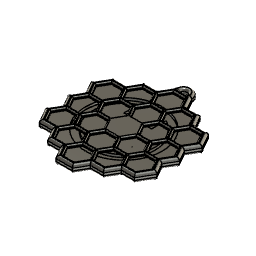
Base-v01 v7 (Autodesk Fusion 360 design; units mm, degrees)
Autodesk Fusion 360 part; units mm, degrees
sketch "Skizze1" plane through (0, 0, 0) normal (0, 0, 1) x (1, 0, 0)
  line L0 (2.5981, -13.5) -> (5.1962, -9) construction
  line L1 (5.1962, -9) -> (2.5981, -4.5) construction
  line L2 (2.5981, -4.5) -> (-2.5981, -4.5) construction
  line L3 (-2.5981, -4.5) -> (-5.1962, -9) construction
  line L4 (-5.1962, -9) -> (-2.5981, -13.5) construction
  line L5 (-2.5981, -13.5) -> (2.5981, -13.5) construction
  line L6 (-2.5981, -4.5) -> (-5.1962, 0) construction
  line L7 (-5.1962, 0) -> (-10.3923, 0) construction
  line L8 (-10.3923, 0) -> (-12.9904, -4.5) construction
  line L9 (-12.9904, -4.5) -> (-10.3923, -9) construction
  line L10 (-10.3923, -9) -> (-5.1962, -9) construction
  line L11 (-5.1962, -9) -> (-2.5981, -4.5) construction
  line L12 (-5.1962, -9) -> (-10.3923, -9) construction
  line L13 (-10.3923, -9) -> (-12.9904, -13.5) construction
  line L14 (-12.9904, -13.5) -> (-10.3923, -18) construction
  line L15 (-10.3923, -18) -> (-5.1962, -18) construction
  line L16 (-5.1962, -18) -> (-2.5981, -13.5) construction
  line L17 (-2.5981, -13.5) -> (-5.1962, -9) construction
  line L18 (12.9904, -13.5) -> (10.3923, -9) construction
  line L19 (10.3923, -9) -> (5.1962, -9) construction
  line L20 (5.1962, -9) -> (2.5981, -13.5) construction
  line L21 (2.5981, -13.5) -> (5.1962, -18) construction
  line L22 (5.1962, -18) -> (10.3923, -18) construction
  line L23 (10.3923, -18) -> (12.9904, -13.5) construction
  line L24 (12.9904, -4.5) -> (10.3923, 0) construction
  line L25 (10.3923, 0) -> (5.1962, 0) construction
  line L26 (5.1962, 0) -> (2.5981, -4.5) construction
  line L27 (2.5981, -4.5) -> (5.1962, -9) construction
  line L28 (5.1962, -9) -> (10.3923, -9) construction
  line L29 (10.3923, -9) -> (12.9904, -4.5) construction
  line L30 (20.7846, 0) -> (18.1865, 4.5) construction
  line L31 (18.1865, 4.5) -> (12.9904, 4.5) construction
  line L32 (12.9904, 4.5) -> (10.3923, 0) construction
  line L33 (10.3923, 0) -> (12.9904, -4.5) construction
  line L34 (12.9904, -4.5) -> (18.1865, -4.5) construction
  line L35 (18.1865, -4.5) -> (20.7846, 0) construction
  line L36 (10.3923, -9) -> (12.9904, -13.5) construction
  line L37 (12.9904, -13.5) -> (18.1865, -13.5) construction
  line L38 (18.1865, -13.5) -> (20.7846, -9) construction
  line L39 (20.7846, -9) -> (18.1865, -4.5) construction
  line L40 (18.1865, -4.5) -> (12.9904, -4.5) construction
  line L41 (12.9904, -4.5) -> (10.3923, -9) construction
  line L42 (-5.1962, 0) -> (-2.5981, -4.5) construction
  line L43 (-2.5981, -4.5) -> (2.5981, -4.5) construction
  line L44 (2.5981, -4.5) -> (5.1962, 0) construction
  line L45 (5.1962, 0) -> (2.5981, 4.5) construction
  line L46 (2.5981, 4.5) -> (-2.5981, 4.5) construction
  line L47 (-2.5981, 4.5) -> (-5.1962, 0) construction
  line L48 (-10.3923, -27) -> (-5.1962, -27) construction
  line L49 (-5.1962, -27) -> (-2.5981, -22.5) construction
  line L50 (-2.5981, -22.5) -> (-5.1962, -18) construction
  line L51 (-5.1962, -18) -> (-10.3923, -18) construction
  line L52 (-10.3923, -18) -> (-12.9904, -22.5) construction
  line L53 (-12.9904, -22.5) -> (-10.3923, -27) construction
  line L54 (10.3923, -36) -> (12.9904, -31.5) construction
  line L55 (12.9904, -31.5) -> (10.3923, -27) construction
  line L56 (10.3923, -27) -> (5.1962, -27) construction
  line L57 (5.1962, -27) -> (2.5981, -31.5) construction
  line L58 (2.5981, -31.5) -> (5.1962, -36) construction
  line L59 (5.1962, -36) -> (10.3923, -36) construction
  line L60 (2.5981, -31.5) -> (5.1962, -27) construction
  line L61 (5.1962, -27) -> (2.5981, -22.5) construction
  line L62 (2.5981, -22.5) -> (-2.5981, -22.5) construction
  line L63 (-2.5981, -22.5) -> (-5.1962, -27) construction
  line L64 (-5.1962, -27) -> (-2.5981, -31.5) construction
  line L65 (-2.5981, -31.5) -> (2.5981, -31.5) construction
  line L66 (28.5788, -13.5) -> (25.9808, -9) construction
  line L67 (25.9808, -9) -> (20.7846, -9) construction
  line L68 (20.7846, -9) -> (18.1865, -13.5) construction
  line L69 (18.1865, -13.5) -> (20.7846, -18) construction
  line L70 (20.7846, -18) -> (25.9808, -18) construction
  line L71 (25.9808, -18) -> (28.5788, -13.5) construction
  line L72 (12.9904, -22.5) -> (10.3923, -18) construction
  line L73 (10.3923, -18) -> (5.1962, -18) construction
  line L74 (5.1962, -18) -> (2.5981, -22.5) construction
  line L75 (2.5981, -22.5) -> (5.1962, -27) construction
  line L76 (5.1962, -27) -> (10.3923, -27) construction
  line L77 (10.3923, -27) -> (12.9904, -22.5) construction
  line L78 (18.1865, -22.5) -> (12.9904, -22.5) construction
  line L79 (12.9904, -22.5) -> (10.3923, -27) construction
  line L80 (10.3923, -27) -> (12.9904, -31.5) construction
  line L81 (12.9904, -31.5) -> (18.1865, -31.5) construction
  line L82 (18.1865, -31.5) -> (20.7846, -27) construction
  line L83 (20.7846, -27) -> (18.1865, -22.5) construction
  line L84 (10.3923, 9) -> (5.1962, 9) construction
  line L85 (5.1962, 9) -> (2.5981, 4.5) construction
  line L86 (2.5981, 4.5) -> (5.1962, 0) construction
  line L87 (5.1962, 0) -> (10.3923, 0) construction
  line L88 (10.3923, 0) -> (12.9904, 4.5) construction
  line L89 (12.9904, 4.5) -> (10.3923, 9) construction
  line L90 (18.1865, -13.5) -> (12.9904, -13.5) construction
  line L91 (12.9904, -13.5) -> (10.3923, -18) construction
  line L92 (10.3923, -18) -> (12.9904, -22.5) construction
  line L93 (12.9904, -22.5) -> (18.1865, -22.5) construction
  line L94 (18.1865, -22.5) -> (20.7846, -18) construction
  line L95 (20.7846, -18) -> (18.1865, -13.5) construction
  line L96 (25.9808, 0) -> (20.7846, 0) construction
  line L97 (20.7846, 0) -> (18.1865, -4.5) construction
  line L98 (18.1865, -4.5) -> (20.7846, -9) construction
  line L99 (20.7846, -9) -> (25.9808, -9) construction
  line L100 (25.9808, -9) -> (28.5788, -4.5) construction
  line L101 (28.5788, -4.5) -> (25.9808, 0) construction
  line L102 (2.5981, -22.5) -> (5.1962, -18) construction
  line L103 (5.1962, -18) -> (2.5981, -13.5) construction
  line L104 (2.5981, -13.5) -> (-2.5981, -13.5) construction
  line L105 (-2.5981, -13.5) -> (-5.1962, -18) construction
  line L106 (-5.1962, -18) -> (-2.5981, -22.5) construction
  line L107 (-2.5981, -22.5) -> (2.5981, -22.5) construction
  line L108 (28.5788, -22.5) -> (25.9808, -18) construction
  line L109 (25.9808, -18) -> (20.7846, -18) construction
  line L110 (20.7846, -18) -> (18.1865, -22.5) construction
  line L111 (18.1865, -22.5) -> (20.7846, -27) construction
  line L112 (20.7846, -27) -> (25.9808, -27) construction
  line L113 (25.9808, -27) -> (28.5788, -22.5) construction
  line L114 (5.5426, 0.6) -> (10.0459, 0.6)
  line L115 (10.0459, 0.6) -> (12.2976, 4.5)
  line L116 (12.2976, 4.5) -> (10.0459, 8.4)
  line L117 (10.0459, 8.4) -> (5.5426, 8.4)
  line L118 (5.5426, 8.4) -> (3.2909, 4.5)
  line L119 (3.2909, 4.5) -> (5.5426, 0.6)
  line L120 (17.8401, -3.9) -> (20.0918, 0)
  line L121 (20.0918, 0) -> (17.8401, 3.9)
  line L122 (17.8401, 3.9) -> (13.3368, 3.9)
  line L123 (13.3368, 3.9) -> (11.0851, 0)
  line L124 (11.0851, 0) -> (13.3368, -3.9)
  line L125 (13.3368, -3.9) -> (17.8401, -3.9)
  line L126 (25.6344, -8.4) -> (27.886, -4.5)
  line L127 (27.886, -4.5) -> (25.6344, -0.6)
  line L128 (25.6344, -0.6) -> (21.131, -0.6)
  line L129 (21.131, -0.6) -> (18.8794, -4.5)
  line L130 (18.8794, -4.5) -> (21.131, -8.4)
  line L131 (21.131, -8.4) -> (25.6344, -8.4)
  line L132 (17.8401, -12.9) -> (20.0918, -9)
  line L133 (20.0918, -9) -> (17.8401, -5.1)
  line L134 (17.8401, -5.1) -> (13.3368, -5.1)
  line L135 (13.3368, -5.1) -> (11.0851, -9)
  line L136 (11.0851, -9) -> (13.3368, -12.9)
  line L137 (13.3368, -12.9) -> (17.8401, -12.9)
  line L138 (18.8794, -13.5) -> (21.131, -17.4)
  line L139 (21.131, -17.4) -> (25.6344, -17.4)
  line L140 (25.6344, -17.4) -> (27.886, -13.5)
  line L141 (27.886, -13.5) -> (25.6344, -9.6)
  line L142 (25.6344, -9.6) -> (21.131, -9.6)
  line L143 (21.131, -9.6) -> (18.8794, -13.5)
  line L144 (13.3368, -21.9) -> (17.8401, -21.9)
  line L145 (17.8401, -21.9) -> (20.0918, -18)
  line L146 (20.0918, -18) -> (17.8401, -14.1)
  line L147 (17.8401, -14.1) -> (13.3368, -14.1)
  line L148 (13.3368, -14.1) -> (11.0851, -18)
  line L149 (11.0851, -18) -> (13.3368, -21.9)
  line L150 (-2.2517, -12.9) -> (2.2517, -12.9)
  line L151 (2.2517, -12.9) -> (4.5033, -9)
  line L152 (4.5033, -9) -> (2.2517, -5.1)
  line L153 (2.2517, -5.1) -> (-2.2517, -5.1)
  line L154 (-2.2517, -5.1) -> (-4.5033, -9)
  line L155 (-4.5033, -9) -> (-2.2517, -12.9)
  line L156 (-2.2517, -3.9) -> (2.2517, -3.9)
  line L157 (2.2517, -3.9) -> (4.5033, 0)
  line L158 (4.5033, 0) -> (2.2517, 3.9)
  line L159 (2.2517, 3.9) -> (-2.2517, 3.9)
  line L160 (-2.2517, 3.9) -> (-4.5033, 0)
  line L161 (-4.5033, 0) -> (-2.2517, -3.9)
  line L162 (-10.0459, -8.4) -> (-5.5426, -8.4)
  line L163 (-5.5426, -8.4) -> (-3.2909, -4.5)
  line L164 (-3.2909, -4.5) -> (-5.5426, -0.6)
  line L165 (-5.5426, -0.6) -> (-10.0459, -0.6)
  line L166 (-10.0459, -0.6) -> (-12.2976, -4.5)
  line L167 (-12.2976, -4.5) -> (-10.0459, -8.4)
  line L168 (-0.0088, -18) -> (-0.0044, -18.0076)
  line L169 (-0.0044, -18.0076) -> (0.0044, -18.0076)
  line L170 (0.0044, -18.0076) -> (0.0088, -18)
  line L171 (0.0088, -18) -> (0.0044, -17.9924)
  line L172 (0.0044, -17.9924) -> (-0.0044, -17.9924)
  line L173 (-0.0044, -17.9924) -> (-0.0088, -18)
  line L174 (12.2976, -22.5) -> (10.0459, -18.6)
  line L175 (10.0459, -18.6) -> (5.5426, -18.6)
  line L176 (5.5426, -18.6) -> (3.2909, -22.5)
  line L177 (3.2909, -22.5) -> (5.5426, -26.4)
  line L178 (5.5426, -26.4) -> (10.0459, -26.4)
  line L179 (10.0459, -26.4) -> (12.2976, -22.5)
  line L180 (27.886, -22.5) -> (25.6344, -18.6)
  line L181 (25.6344, -18.6) -> (21.131, -18.6)
  line L182 (21.131, -18.6) -> (18.8794, -22.5)
  line L183 (18.8794, -22.5) -> (21.131, -26.4)
  line L184 (21.131, -26.4) -> (25.6344, -26.4)
  line L185 (25.6344, -26.4) -> (27.886, -22.5)
  line L186 (10.0459, -8.4) -> (12.2976, -4.5)
  line L187 (12.2976, -4.5) -> (10.0459, -0.6)
  line L188 (10.0459, -0.6) -> (5.5426, -0.6)
  line L189 (5.5426, -0.6) -> (3.2909, -4.5)
  line L190 (3.2909, -4.5) -> (5.5426, -8.4)
  line L191 (5.5426, -8.4) -> (10.0459, -8.4)
  line L192 (-5.5426, -26.4) -> (-3.2909, -22.5)
  line L193 (-3.2909, -22.5) -> (-5.5426, -18.6)
  line L194 (-5.5426, -18.6) -> (-10.0459, -18.6)
  line L195 (-10.0459, -18.6) -> (-12.2976, -22.5)
  line L196 (-12.2976, -22.5) -> (-10.0459, -26.4)
  line L197 (-10.0459, -26.4) -> (-5.5426, -26.4)
  line L198 (2.2517, -30.9) -> (4.5033, -27)
  line L199 (4.5033, -27) -> (2.2517, -23.1)
  line L200 (2.2517, -23.1) -> (-2.2517, -23.1)
  line L201 (-2.2517, -23.1) -> (-4.5033, -27)
  line L202 (-4.5033, -27) -> (-2.2517, -30.9)
  line L203 (-2.2517, -30.9) -> (2.2517, -30.9)
  line L204 (12.2976, -31.5) -> (10.0459, -27.6)
  line L205 (10.0459, -27.6) -> (5.5426, -27.6)
  line L206 (5.5426, -27.6) -> (3.2909, -31.5)
  line L207 (3.2909, -31.5) -> (5.5426, -35.4)
  line L208 (5.5426, -35.4) -> (10.0459, -35.4)
  line L209 (10.0459, -35.4) -> (12.2976, -31.5)
  line L210 (20.0918, -27) -> (17.8401, -23.1)
  line L211 (17.8401, -23.1) -> (13.3368, -23.1)
  line L212 (13.3368, -23.1) -> (11.0851, -27)
  line L213 (11.0851, -27) -> (13.3368, -30.9)
  line L214 (13.3368, -30.9) -> (17.8401, -30.9)
  line L215 (17.8401, -30.9) -> (20.0918, -27)
  line L216 (-2.2517, -21.9) -> (2.2517, -21.9)
  line L217 (2.2517, -21.9) -> (4.5033, -18)
  line L218 (4.5033, -18) -> (2.2517, -14.1)
  line L219 (2.2517, -14.1) -> (-2.2517, -14.1)
  line L220 (-2.2517, -14.1) -> (-4.5033, -18)
  line L221 (-4.5033, -18) -> (-2.2517, -21.9)
  line L222 (-10.0459, -17.4) -> (-5.5426, -17.4)
  line L223 (-5.5426, -17.4) -> (-3.2909, -13.5)
  line L224 (-3.2909, -13.5) -> (-5.5426, -9.6)
  line L225 (-5.5426, -9.6) -> (-10.0459, -9.6)
  line L226 (-10.0459, -9.6) -> (-12.2976, -13.5)
  line L227 (-12.2976, -13.5) -> (-10.0459, -17.4)
  line L228 (13.6832, 5.7) -> (11.0851, 10.2)
  line L229 (11.0851, 10.2) -> (4.5033, 10.2)
  line L230 (4.5033, 10.2) -> (1.9053, 5.7)
  line L231 (1.9053, 5.7) -> (-3.2909, 5.7)
  line L232 (-3.2909, 5.7) -> (-5.889, 1.2)
  line L233 (-5.889, 1.2) -> (-11.0851, 1.2)
  line L234 (-11.0851, 1.2) -> (-14.376, -4.5)
  line L235 (-14.376, -4.5) -> (-11.7779, -9)
  line L236 (-11.7779, -9) -> (-14.376, -13.5)
  line L237 (-14.376, -13.5) -> (-11.7779, -18)
  line L238 (-11.7779, -18) -> (-14.376, -22.5)
  line L239 (-14.376, -22.5) -> (-11.0851, -28.2)
  line L240 (-11.0851, -28.2) -> (-5.889, -28.2)
  line L241 (-5.889, -28.2) -> (-3.2909, -32.7)
  line L242 (-3.2909, -32.7) -> (1.9053, -32.7)
  line L243 (1.9053, -32.7) -> (4.5033, -37.2)
  line L244 (4.5033, -37.2) -> (11.0851, -37.2)
  line L245 (11.0851, -37.2) -> (13.6832, -32.7)
  line L246 (13.6832, -32.7) -> (18.8794, -32.7)
  line L247 (18.8794, -32.7) -> (21.4774, -28.2)
  line L248 (21.4774, -28.2) -> (26.6736, -28.2)
  line L249 (26.6736, -28.2) -> (29.9645, -22.5)
  line L250 (29.9645, -22.5) -> (27.3664, -18)
  line L251 (27.3664, -18) -> (29.9645, -13.5)
  line L252 (29.9645, -13.5) -> (27.3664, -9)
  line L253 (27.3664, -9) -> (29.9645, -4.5)
  line L254 (29.9645, -4.5) -> (26.6736, 1.2)
  line L255 (26.6736, 1.2) -> (21.4774, 1.2)
  line L256 (21.4774, 1.2) -> (18.8794, 5.7)
  line L257 (18.8794, 5.7) -> (13.6832, 5.7)
  arc A0 (11.0851, 10.2) -> (4.5033, 10.2) centre (7.7942, 10.2) ccw
  arc A1 (9.2851, 10.2) -> (6.3033, 10.2) centre (7.7942, 10.2) ccw
  point P0 (0, -9)
  point P1 (-7.7942, -4.5)
  point P2 (-7.7942, -13.5)
  point P3 (7.7942, -13.5)
  point P4 (7.7942, -4.5)
  point P5 (15.5885, 0)
  point P6 (15.5885, -9)
  point P7 (-7.7942, -22.5)
  point P8 (7.7942, -31.5)
  point P9 (0, -27)
  point P10 (23.3827, -13.5)
  point P11 (7.7942, -22.5)
  point P12 (15.5885, -27)
  point P13 (7.7942, 4.5)
  point P14 (15.5885, -18)
  point P15 (23.3827, -4.5)
  point P16 (0, -18)
  point P17 (23.3827, -22.5)
  point P18 (7.7942, 4.5)
  point P19 (15.5885, 0)
  point P20 (23.3827, -4.5)
  point P21 (15.5885, -9)
  point P22 (23.3827, -13.5)
  point P23 (15.5885, -18)
  point P24 (7.7942, -13.5)
  point P25 (0, -9)
  point P26 (-7.7942, -4.5)
  point P27 (-7.7942, -13.5)
  point P28 (0, -18)
  point P29 (7.7942, -22.5)
  point P30 (23.3827, -22.5)
  point P31 (7.7942, -4.5)
  point P32 (-7.7942, -22.5)
  point P33 (0, -27)
  point P34 (7.7942, -31.5)
  point P35 (15.5885, -27)
  point P36 (0, -18)
  point P37 (-7.7942, -13.5)
  point P38 (7.7942, 10.2)
  point P39 (7.7942, 8.4)
  dimension "d1" = 9
  dimension "d2" = 7.8
  dimension "d3" = 1.2
  dimension "d8" = 47.4
  dimension "d9" = -1.8
  constraint horizontal L2
  constraint equal L40 L45
  constraint equal L32 L45
  constraint equal L26 L40
  constraint equal L2 L40
  constraint equal L19 L40
  constraint equal L13 L46
  constraint equal L7 L46
  constraint equal L46 L103
  constraint equal L46 L55
  constraint equal L46 L50
  constraint equal L45 L61
  constraint equal L44 L67
  constraint equal L44 L73
  constraint equal L44 L79
  constraint equal L44 L85
  constraint equal L44 L91
  constraint equal L44 L97
  constraint horizontal L51
  constraint horizontal L46
  constraint horizontal L40
  constraint horizontal L31
  constraint horizontal L25
  constraint horizontal L7
  constraint horizontal L56
  constraint horizontal L104
  constraint horizontal L19
  constraint horizontal L96
  constraint horizontal L90
  constraint horizontal L84
  constraint horizontal L78
  constraint horizontal L73
  constraint horizontal L67
  constraint horizontal L62
  constraint midpoint L6 L42
  constraint midpoint L2 L43
  constraint midpoint L26 L44
  constraint midpoint L29 L41
  constraint midpoint L19 L28
  constraint midpoint L34 L40
  constraint midpoint L35 L97
  constraint midpoint L37 L90
  constraint midpoint L5 L104
  constraint midpoint L22 L73
  constraint horizontal L12
  constraint midpoint L10 L12
  constraint midpoint L25 L87
  constraint midpoint L15 L51
  constraint midpoint L62 L107
  constraint midpoint L56 L76
  constraint midpoint L78 L93
  constraint midpoint L67 L99
  constraint equal L46 L109
  constraint horizontal L109
  constraint midpoint L70 L109
  constraint coincident P18 P13
  constraint coincident P19 P5
  constraint coincident P20 P15
  constraint coincident P21 P6
  constraint coincident P22 P10
  constraint coincident P23 P14
  constraint coincident P24 P3
  constraint coincident P25 P0
  constraint coincident P26 P1
  constraint coincident P37 P27
  constraint coincident P36 P28
  constraint coincident P29 P11
  constraint coincident P30 P17
  constraint coincident P31 P4
  constraint coincident P32 P7
  constraint coincident P33 P9
  constraint coincident P34 P8
  constraint coincident P35 P12
  constraint horizontal L117
  constraint horizontal L122
  constraint horizontal L128
  constraint horizontal L134
  constraint horizontal L142
  constraint horizontal L181
  constraint horizontal L147
  constraint horizontal L211
  constraint horizontal L205
  constraint horizontal L175
  constraint horizontal L188
  constraint horizontal L153
  constraint horizontal L169
  constraint horizontal L200
  constraint horizontal L194
  constraint horizontal L165
  constraint horizontal L219
  constraint horizontal L225
  constraint horizontal L159
  constraint equal L117 L122
  constraint equal L122 L159
  constraint equal L114 L188
  constraint equal L120 L128
  constraint equal L125 L134
  constraint equal L131 L142
  constraint equal L137 L147
  constraint equal L152 L190
  constraint equal L161 L164
  constraint equal L162 L225
  constraint equal L150 L219
  constraint equal L194 L222
  constraint equal L200 L216
  constraint equal L178 L205
  constraint equal L144 L211
  constraint equal L139 L181
  constraint equal L175 L188
  constraint midpoint L117 P39
  constraint midpoint L229 P38
  constraint coincident P38 A0.centre
  measures "d1" distance of L42 L45
  measures "d2" distance of L116 L119
  measures "d8" distance of L229 L244
extrude "Extrusion1" add sketch "Skizze1" along normal blind 1 contours L228 L229 L230 L231 L232 L233 L234 L235 L236 L237 L238 L239 L240 L241 L242 L243 L244 L245 L246 L247 L248 L249 L250 L251 L252 L253 L254 L255 L256 L257 | L229 A0 A1
sketch "Skizze2" plane through (0, 0, 0) normal (0, 0, -1) x (1, 0, 0)
  arc A0 (6.3033, -10.2) -> (9.2851, -10.2) centre (7.7942, -10.2) ccw
  line L0 (6.3033, -10.2) -> (9.2851, -10.2)
  arc A1 (4.5033, -10.2) -> (11.0851, -10.2) centre (7.7942, -10.2) ccw
  line L1 (11.0851, -10.2) -> (13.6832, -5.7)
  line L2 (13.6832, -5.7) -> (18.8794, -5.7)
  line L3 (18.8794, -5.7) -> (21.4774, -1.2)
  line L4 (21.4774, -1.2) -> (26.6736, -1.2)
  line L5 (26.6736, -1.2) -> (29.9645, 4.5)
  line L6 (29.9645, 4.5) -> (27.3664, 9)
  line L7 (27.3664, 9) -> (29.9645, 13.5)
  line L8 (29.9645, 13.5) -> (27.3664, 18)
  line L9 (27.3664, 18) -> (29.9645, 22.5)
  line L10 (29.9645, 22.5) -> (26.6736, 28.2)
  line L11 (26.6736, 28.2) -> (21.4774, 28.2)
  line L12 (21.4774, 28.2) -> (18.8794, 32.7)
  line L13 (18.8794, 32.7) -> (13.6832, 32.7)
  line L14 (13.6832, 32.7) -> (11.0851, 37.2)
  line L15 (11.0851, 37.2) -> (4.5033, 37.2)
  line L16 (4.5033, 37.2) -> (1.9053, 32.7)
  line L17 (1.9053, 32.7) -> (-3.2909, 32.7)
  line L18 (-3.2909, 32.7) -> (-5.889, 28.2)
  line L19 (-5.889, 28.2) -> (-11.0851, 28.2)
  line L20 (-11.0851, 28.2) -> (-14.376, 22.5)
  line L21 (-14.376, 22.5) -> (-11.7779, 18)
  line L22 (-11.7779, 18) -> (-14.376, 13.5)
  line L23 (-14.376, 13.5) -> (-11.7779, 9)
  line L24 (-11.7779, 9) -> (-14.376, 4.5)
  line L25 (-14.376, 4.5) -> (-11.0851, -1.2)
  line L26 (-11.0851, -1.2) -> (-5.889, -1.2)
  line L27 (-5.889, -1.2) -> (-3.2909, -5.7)
  line L28 (-3.2909, -5.7) -> (1.9053, -5.7)
  line L29 (1.9053, -5.7) -> (4.5033, -10.2)
  line L30 (12.9904, 13.5) -> (10.3923, 18) construction
  line L31 (-10.3923, 18) -> (-12.9904, 13.5) construction
  line L32 (-5.1962, 9) -> (-10.3923, 9) construction
  line L33 (-2.5981, 22.5) -> (2.5981, 22.5) construction
  line L34 (25.9808, 18) -> (20.7846, 18) construction
  line L35 (15.5841, 17.9924) -> (15.5929, 17.9924)
  line L36 (2.5981, 13.5) -> (-2.5981, 13.5) construction
  line L37 (20.7846, 27) -> (18.1865, 31.5) construction
  line L38 (21.4774, 28.2) -> (18.8794, 32.7)
  line L39 (-12.9904, 4.5) -> (-10.3923, 0) construction
  line L40 (-10.3923, 0) -> (-5.1962, 0) construction
  line L41 (13.6832, 32.7) -> (11.0851, 37.2)
  line L42 (5.1962, 9) -> (2.5981, 13.5) construction
  line L43 (25.9808, 18) -> (28.5788, 22.5) construction
  line L44 (27.3664, 18) -> (29.9645, 22.5)
  line L45 (-5.889, -1.2) -> (-3.2909, -5.7)
  line L46 (-5.1962, 27) -> (-2.5981, 22.5) construction
  line L47 (-5.1962, 0) -> (-2.5981, 4.5) construction
  line L48 (2.5981, 4.5) -> (5.1962, 0) construction
  line L49 (15.5841, 18.0076) -> (15.5797, 18)
  line L50 (2.5981, 13.5) -> (5.1962, 9) construction
  line L51 (15.5973, 18) -> (15.5929, 18.0076)
  line L52 (20.7846, 18) -> (25.9808, 18) construction
  line L53 (-3.2909, -5.7) -> (1.9053, -5.7)
  line L54 (26.6736, 28.2) -> (21.4774, 28.2)
  line L55 (-2.5981, 4.5) -> (2.5981, 4.5) construction
  line L56 (25.9808, 27) -> (20.7846, 27) construction
  line L57 (12.9904, 22.5) -> (18.1865, 22.5) construction
  line L58 (18.1865, 31.5) -> (12.9904, 31.5) construction
  line L59 (5.1962, 27) -> (2.5981, 31.5) construction
  line L60 (18.1865, 22.5) -> (12.9904, 22.5) construction
  line L61 (18.8794, 32.7) -> (13.6832, 32.7)
  line L62 (15.5929, 17.9924) -> (15.5973, 18)
  line L63 (-14.376, 13.5) -> (-11.7779, 9)
  line L64 (-3.2909, 32.7) -> (-5.889, 28.2)
  line L65 (-12.9904, 13.5) -> (-10.3923, 9) construction
  line L66 (5.1962, 0) -> (2.5981, -4.5) construction
  line L67 (10.3923, 36) -> (5.1962, 36) construction
  line L68 (-2.5981, 31.5) -> (-5.1962, 27) construction
  line L69 (-5.1962, 9) -> (-2.5981, 4.5) construction
  line L70 (-2.5981, 22.5) -> (-5.1962, 18) construction
  line L71 (29.9645, 22.5) -> (26.6736, 28.2)
  line L72 (-5.1962, 0) -> (-2.5981, -4.5) construction
  line L73 (15.5929, 18.0076) -> (15.5841, 18.0076)
  line L74 (5.1962, 9) -> (2.5981, 4.5) construction
  line L75 (-2.5981, 13.5) -> (2.5981, 13.5) construction
  line L76 (10.3923, 18) -> (12.9904, 22.5) construction
  line L77 (10.3923, 27) -> (5.1962, 27) construction
  line L78 (20.7846, 9) -> (18.1865, 4.5) construction
  line L79 (18.1865, 22.5) -> (20.7846, 27) construction
  line L80 (28.5788, 4.5) -> (25.9808, 9) construction
  line L81 (12.9904, 4.5) -> (10.3923, 9) construction
  line L82 (15.5797, 18) -> (15.5841, 17.9924)
  line L83 (10.3923, 9) -> (12.9904, 4.5) construction
  line L84 (5.1962, -9) -> (10.3923, -9) construction
  line L85 (-10.3923, 9) -> (-12.9904, 4.5) construction
  line L86 (18.1865, 4.5) -> (20.7846, 9) construction
  line L87 (20.7846, 27) -> (18.1865, 22.5) construction
  arc A2 (4.5033, -10.2) -> (11.0851, -10.2) centre (7.7942, -10.2) ccw
  line L88 (12.9904, 31.5) -> (10.3923, 27) construction
  line L89 (5.1962, 27) -> (10.3923, 27) construction
  line L90 (2.5981, 4.5) -> (5.1962, 9) construction
  line L91 (5.1962, 0) -> (10.3923, 0) construction
  line L92 (-11.7779, 9) -> (-14.376, 4.5)
  line L93 (-5.1962, 18) -> (-2.5981, 22.5) construction
  line L94 (4.5033, -10.2) -> (11.0851, -10.2)
  line L95 (-2.5981, 4.5) -> (-5.1962, 9) construction
  line L96 (-2.5981, 22.5) -> (-5.1962, 27) construction
  line L97 (28.5788, 22.5) -> (25.9808, 27) construction
  line L98 (5.1962, 27) -> (2.5981, 22.5) construction
  line L99 (4.5033, 37.2) -> (1.9053, 32.7)
  line L100 (-11.0851, -1.2) -> (-5.889, -1.2)
  line L101 (5.1962, 36) -> (2.5981, 31.5) construction
  line L102 (-2.5981, -4.5) -> (2.5981, -4.5) construction
  line L103 (2.5981, 4.5) -> (-2.5981, 4.5) construction
  line L104 (-10.3923, 27) -> (-12.9904, 22.5) construction
  line L105 (-12.9904, 22.5) -> (-10.3923, 18) construction
  arc A3 (6.3033, -10.2) -> (9.2851, -10.2) centre (7.7942, -10.2) ccw
  line L106 (2.5981, -4.5) -> (5.1962, -9) construction
  line L107 (5.1962, 0) -> (2.5981, 4.5) construction
  line L108 (-2.5981, 4.5) -> (-5.1962, 0) construction
  line L109 (2.5981, 22.5) -> (-2.5981, 22.5) construction
  line L110 (1.9053, -5.7) -> (4.5033, -10.2)
  line L111 (2.5981, 31.5) -> (5.1962, 27) construction
  line L112 (2.5981, -4.5) -> (5.1962, 0) construction
  line L113 (-5.1962, 9) -> (-2.5981, 13.5) construction
  line L114 (-5.889, 28.2) -> (-11.0851, 28.2)
  line L115 (2.5981, 31.5) -> (-2.5981, 31.5) construction
  line L116 (20.7846, 18) -> (18.1865, 22.5) construction
  line L117 (1.9053, 32.7) -> (-3.2909, 32.7)
  line L118 (-10.3923, 18) -> (-5.1962, 18) construction
  line L119 (-11.0851, 28.2) -> (-14.376, 22.5)
  line L120 (18.1865, 22.5) -> (20.7846, 18) construction
  line L121 (-10.3923, 9) -> (-5.1962, 9) construction
  line L122 (-2.5981, 13.5) -> (-5.1962, 9) construction
  line L123 (-5.1962, 27) -> (-10.3923, 27) construction
  line L124 (-14.376, 22.5) -> (-11.7779, 18)
  line L125 (2.5981, 22.5) -> (5.1962, 27) construction
  line L126 (2.5981, 22.5) -> (5.1962, 18) construction
  line L127 (-5.1962, 18) -> (-10.3923, 18) construction
  line L128 (-14.376, 4.5) -> (-11.0851, -1.2)
  line L129 (5.1962, 18) -> (2.5981, 22.5) construction
  line L130 (18.1865, 13.5) -> (20.7846, 18) construction
  line L131 (12.9904, 22.5) -> (10.3923, 27) construction
  line L132 (5.1962, 9) -> (10.3923, 9) construction
  line L133 (10.3923, 0) -> (5.1962, 0) construction
  line L134 (5.1962, 18) -> (10.3923, 18) construction
  line L135 (11.0851, 37.2) -> (4.5033, 37.2)
  line L136 (12.9904, 22.5) -> (10.3923, 18) construction
  line L137 (10.3923, 18) -> (5.1962, 18) construction
  line L138 (18.1865, 13.5) -> (12.9904, 13.5) construction
  line L139 (20.7846, 18) -> (18.1865, 13.5) construction
  line L140 (10.3923, 27) -> (12.9904, 22.5) construction
  line L141 (10.3923, 9) -> (12.9904, 13.5) construction
  line L142 (5.1962, 18) -> (2.5981, 13.5) construction
  line L143 (10.3923, 18) -> (12.9904, 13.5) construction
  line L144 (12.9904, 13.5) -> (10.3923, 9) construction
  line L145 (10.3923, 9) -> (5.1962, 9) construction
  line L146 (10.3923, 27) -> (12.9904, 31.5) construction
  line L147 (12.9904, 13.5) -> (18.1865, 13.5) construction
  line L148 (29.9645, 4.5) -> (27.3664, 9)
  line L149 (12.9904, 31.5) -> (10.3923, 36) construction
  line L150 (20.7846, 9) -> (25.9808, 9) construction
  line L151 (28.5788, 13.5) -> (25.9808, 18) construction
  line L152 (-2.5981, 13.5) -> (-5.1962, 18) construction
  line L153 (18.1865, 13.5) -> (20.7846, 9) construction
  line L154 (25.9808, 9) -> (28.5788, 13.5) construction
  line L155 (29.9645, 13.5) -> (27.3664, 18)
  line L156 (-5.1962, 18) -> (-2.5981, 13.5) construction
  line L157 (20.7846, 9) -> (18.1865, 13.5) construction
  line L158 (27.3664, 9) -> (29.9645, 13.5)
  line L159 (25.9808, 9) -> (20.7846, 9) construction
  line L160 (-11.7779, 18) -> (-14.376, 13.5)
  line L161 (2.5981, 13.5) -> (5.1962, 18) construction
  line L162 (12.9904, -4.5) -> (18.1865, -4.5) construction
  line L163 (13.6832, -5.7) -> (18.8794, -5.7)
  line L164 (18.1865, 4.5) -> (12.9904, 4.5) construction
  line L165 (25.9808, 0) -> (28.5788, 4.5) construction
  line L166 (10.3923, 0) -> (12.9904, 4.5) construction
  line L167 (18.1865, -4.5) -> (20.7846, 0) construction
  line L168 (11.0851, -10.2) -> (13.6832, -5.7)
  line L169 (10.3923, 0) -> (12.9904, -4.5) construction
  line L170 (20.7846, 0) -> (18.1865, 4.5) construction
  line L171 (26.6736, -1.2) -> (29.9645, 4.5)
  line L172 (12.9904, -4.5) -> (10.3923, 0) construction
  line L173 (12.9904, 4.5) -> (10.3923, 0) construction
  line L174 (18.1865, 4.5) -> (20.7846, 0) construction
  line L175 (18.8794, -5.7) -> (21.4774, -1.2)
  line L176 (12.9904, 4.5) -> (18.1865, 4.5) construction
  line L177 (10.3923, -9) -> (12.9904, -4.5) construction
  line L178 (20.7846, 0) -> (25.9808, 0) construction
  line L179 (21.4774, -1.2) -> (26.6736, -1.2)
  circle A4 centre (7.7942, 13.5) radius 15.25
  circle A5 centre (7.7942, 13.5) radius 12.5
  line L180 (20.2942, 13.5) -> (-4.7058, 13.5)
  line L181 (13.2942, 2.275) -> (13.2942, 8)
  line L182 (13.2942, 8) -> (2.2942, 8)
  line L183 (2.2942, 8) -> (2.2942, 2.275)
  line L184 (7.7942, 13.5) -> (7.7942, 1) construction
  point P0 (0, 9)
  point P1 (7.7942, 4.5)
  point P2 (7.7942, 13.5)
  point P3 (23.3827, 4.5)
  point P4 (15.5885, 0)
  point P5 (23.3827, 22.5)
  point P6 (15.5885, 9)
  point P7 (23.3827, 13.5)
  point P8 (23.3827, 13.5)
  point P9 (7.7942, -4.5)
  point P10 (15.5885, 9)
  point P11 (7.7942, 13.5)
  point P12 (-7.7942, 4.5)
  point P13 (-7.7942, 13.5)
  point P14 (0, 9)
  point P15 (0, 18)
  point P16 (15.5885, 0)
  point P17 (23.3827, 4.5)
  point P18 (23.3827, 22.5)
  point P19 (-7.7942, 22.5)
  point P20 (15.5885, 27)
  point P21 (15.5885, 18)
  point P22 (15.5885, 0)
  point P23 (7.7942, 31.5)
  point P24 (7.7942, 22.5)
  point P25 (7.7942, 4.5)
  point P26 (0, 27)
  point P27 (7.7942, -10.2)
  point P28 (7.7942, -8.4)
  point P29 (23.3827, 13.5)
  point P30 (15.5885, 18)
  point P31 (-7.7942, 22.5)
  point P32 (7.7942, 22.5)
  point P33 (-7.7942, 4.5)
  point P34 (7.7942, -4.5)
  point P35 (0, 18)
  point P36 (7.7942, 31.5)
  point P37 (0, 27)
  point P38 (15.5885, 27)
  point P39 (-7.7942, 13.5)
  point P40 (15.5885, 18)
  point P41 (7.7942, 8)
  dimension "d12" = 9
  dimension "d14" = 47.4
  dimension "d15" = 30.5
  dimension "d16" = 25
  dimension "d41" = 7
  dimension "d42" = 11
  constraint equal L55 L169
  constraint equal L112 L169
  constraint equal L55 L166
  constraint equal L55 L176
  constraint equal L55 L132
  constraint equal L154 L162
  constraint equal L162 L178
  constraint equal L143 L162
  constraint equal L111 L162
  constraint equal L120 L162
  constraint equal L140 L169
  constraint equal L121 L173
  constraint equal L134 L173
  constraint equal L125 L173
  constraint equal L173 L177
  constraint equal L161 L173
  constraint equal L47 L173
  constraint midpoint L170 L174
  constraint midpoint L164 L176
  constraint midpoint L166 L173
  constraint midpoint L74 L90
  constraint midpoint L132 L145
  constraint midpoint L55 L103
  constraint midpoint L47 L108
  constraint midpoint L36 L75
  constraint midpoint L138 L147
  constraint midpoint L134 L137
  constraint midpoint L150 L159
  constraint midpoint L91 L133
  constraint coincident P22 P16
  constraint midpoint L34 L52
  constraint midpoint L57 L60
  constraint midpoint L77 L89
  constraint midpoint L33 L109
  constraint midpoint L32 L121
  constraint equal L118 L162
  constraint midpoint L118 L127
  constraint coincident P34 P9
  constraint coincident P33 P12
  constraint coincident P14 P0
  constraint coincident P39 P13
  constraint coincident P35 P15
  constraint coincident P11 P2
  constraint coincident P10 P6
  constraint coincident P17 P3
  constraint coincident P29 P8
  constraint coincident P40 P30
  constraint coincident P32 P24
  constraint coincident P31 P19
  constraint coincident P25 P1
  constraint coincident P18 P5
  constraint coincident P38 P20
  constraint coincident P36 P23
  constraint coincident P37 P26
  constraint midpoint P27 L94
  constraint coincident P27 A0.centre
  constraint parallel L106 L110
  constraint parallel L84 L94
  constraint parallel L168 L177
  constraint parallel L162 L163
  constraint parallel L167 L175
  constraint parallel L178 L179
  constraint parallel L165 L171
  constraint parallel L80 L148
  constraint parallel L154 L158
  constraint parallel L151 L155
  constraint parallel L43 L44
  constraint parallel L71 L97
  constraint parallel L54 L56
  constraint parallel L37 L38
  constraint parallel L58 L61
  constraint parallel L41 L149
  constraint parallel L67 L135
  constraint parallel L99 L101
  constraint parallel L115 L117
  constraint parallel L64 L68
  constraint parallel L114 L123
  constraint parallel L104 L119
  constraint parallel L105 L124
  constraint parallel L31 L160
  constraint parallel L63 L65
  constraint parallel L85 L92
  constraint parallel L39 L128
  constraint parallel L40 L100
  constraint parallel L45 L72
  constraint parallel L53 L102
  constraint concentric A2 A3
  constraint concentric A4 A5
  constraint midpoint P11 L180
  constraint coincident A5 L180.start
  constraint coincident A5 L181.start
  constraint coincident A5 L183.end
  constraint horizontal L182
  constraint vertical L181
  constraint vertical L183
  constraint coincident A5 L184.end
  constraint vertical L184
  constraint midpoint L182 P41
  constraint coincident L184 P41
  measures "d12" distance of L169 L170
  measures "d14" distance of L94 L135
  measures "d15" diameter of A4
  measures "d16" diameter of A5
  measures "d41" distance of L182 L184.end
  measures "d42" distance of L181 L183
extrude "Extrusion3" add sketch "Skizze2" along normal blind 2 contours L0 L1 L2 L3 L4 L5 L6 L7 L8 L9 L10 L11 L12 L13 L14 L15 L16 L17 L18 L19 L20 L21 L22 L23 L24 L25 L26 L27 L28 L29 L38 L41 L44 L45 L53 L54 L61 L63 L64 L71 L92 L94 L99 L100 L110 L114 L117 L119 L124 L128 L135 L148 L155 L158 L160 L163 L168 L171 L175 L179 | A0 A1 A2 L94 A3 | A4 | A5 L180 | A5 L180 L181 L182 L183 | A5 L181 L182 L183
extrude "Extrusion4" cut sketch "Skizze2" along normal blind 1 contours A4 | A5 L181 L182 L183
fillet "Abrundung1" radius 1 64 edges at (12.3842, -34.95, -2) (16.2813, -32.7, -2) (20.1784, -30.45, -2) (24.0755, -28.2, -2) (28.319, -25.35, -2) (28.6654, -20.25, -2) (28.6654, -15.75, -2) (28.6654, -11.25, -2) (28.6654, -6.75, -2) (28.319, -1.65, -2) (24.0755, 1.2, -2) (20.1784, 3.45, -2) (16.2813, 5.7, -2) (12.3842, 7.95, -2) (7.7942, 13.4909, -2) (3.2043, 7.95, -2) (7.7942, 10.2, -2) (7.7942, 11.6909, -2) (-0.6928, 5.7, -2) (-4.5899, 3.45, -2) (-8.487, 1.2, -2) (-12.7306, -1.65, -2) (-13.077, -6.75, -2) (-13.077, -11.25, -2) (-13.077, -15.75, -2) (-13.077, -20.25, -2) (-12.7306, -25.35, -2) (-8.487, -28.2, -2) (7.7942, -37.2, -2) (3.2043, -34.95, -2) (-0.6928, -32.7, -2) (-4.5899, -30.45, -2) (7.7942, 10.2, 1) (7.7942, 11.6909, 1) (7.7942, 13.4909, 1) (3.2043, 7.95, 1) (-0.6928, 5.7, 1) (-4.5899, 3.45, 1) (-8.487, 1.2, 1) (-12.7306, -1.65, 1) (-13.077, -6.75, 1) (-13.077, -11.25, 1) (-13.077, -15.75, 1) (-13.077, -20.25, 1) (-12.7306, -25.35, 1) (-8.487, -28.2, 1) (-4.5899, -30.45, 1) (-0.6928, -32.7, 1) (3.2043, -34.95, 1) (7.7942, -37.2, 1) (12.3842, -34.95, 1) (16.2813, -32.7, 1) (20.1784, -30.45, 1) (24.0755, -28.2, 1) (28.319, -25.35, 1) (28.6654, -20.25, 1) (28.6654, -15.75, 1) (28.6654, -11.25, 1) (28.6654, -6.75, 1) (28.319, -1.65, 1) (24.0755, 1.2, 1) (20.1784, 3.45, 1) (16.2813, 5.7, 1) (12.3842, 7.95, 1)
fillet "Abrundung2" radius 0.5 108 edges at (11.1717, 2.55, 1) (7.7942, 0.6, 1) (4.4167, 2.55, 1) (4.4167, 6.45, 1) (7.7942, 8.4, 1) (11.1717, 6.45, 1) (12.211, 1.95, 1) (15.5885, 3.9, 1) (18.966, 1.95, 1) (18.966, -1.95, 1) (15.5885, -3.9, 1) (12.211, -1.95, 1) (20.0052, -6.45, 1) (23.3827, -8.4, 1) (26.7602, -6.45, 1) (26.7602, -2.55, 1) (23.3827, -0.6, 1) (20.0052, -2.55, 1) (26.7602, -11.55, 1) (26.7602, -15.45, 1) (23.3827, -17.4, 1) (20.0052, -15.45, 1) (20.0052, -11.55, 1) (23.3827, -9.6, 1) (18.966, -10.95, 1) (18.966, -7.05, 1) (15.5885, -5.1, 1) (12.211, -7.05, 1) (12.211, -10.95, 1) (15.5885, -12.9, 1) (11.1717, -6.45, 1) (11.1717, -2.55, 1) (7.7942, -0.6, 1) (4.4167, -2.55, 1) (4.4167, -6.45, 1) (7.7942, -8.4, 1) (3.3775, -1.95, 1) (0, -3.9, 1) (-3.3775, -1.95, 1) (-3.3775, 1.95, 1) (0, 3.9, 1) (3.3775, 1.95, 1) (3.3775, -10.95, 1) (3.3775, -7.05, 1) (0, -12.9, 1) (-3.3775, -10.95, 1) (-3.3775, -7.05, 1) (0, -5.1, 1) (-4.4167, -6.45, 1) (-4.4167, -2.55, 1) (-7.7942, -0.6, 1) (-11.1717, -2.55, 1) (-11.1717, -6.45, 1) (-7.7942, -8.4, 1) (-4.4167, -11.55, 1) (-4.4167, -15.45, 1) (-7.7942, -17.4, 1) (-11.1717, -15.45, 1) (-11.1717, -11.55, 1) (-7.7942, -9.6, 1) (-4.4167, -24.45, 1) (-4.4167, -20.55, 1) (-7.7942, -18.6, 1) (-11.1717, -20.55, 1) (-11.1717, -24.45, 1) (-7.7942, -26.4, 1) (0, -21.9, 1) (3.3775, -19.95, 1) (3.3775, -16.05, 1) (0, -14.1, 1) (-3.3775, -16.05, 1) (-3.3775, -19.95, 1) (3.3775, -28.95, 1) (3.3775, -25.05, 1) (0, -23.1, 1) (-3.3775, -25.05, 1) (-3.3775, -28.95, 1) (0, -30.9, 1) (4.4167, -29.55, 1) (7.7942, -27.6, 1) (11.1717, -29.55, 1) (11.1717, -33.45, 1) (7.7942, -35.4, 1) (4.4167, -33.45, 1) (15.5885, -30.9, 1) (18.966, -28.95, 1) (18.966, -25.05, 1) (15.5885, -23.1, 1) (12.211, -25.05, 1) (12.211, -28.95, 1) (11.1717, -24.45, 1) (7.7942, -26.4, 1) (11.1717, -20.55, 1) (7.7942, -18.6, 1) (4.4167, -20.55, 1) (4.4167, -24.45, 1) (12.211, -19.95, 1) (15.5885, -21.9, 1) (18.966, -19.95, 1) (18.966, -16.05, 1) (15.5885, -14.1, 1) (12.211, -16.05, 1) (20.0052, -20.55, 1) (20.0052, -24.45, 1) (23.3827, -26.4, 1) (26.7602, -24.45, 1) (26.7602, -20.55, 1) (23.3827, -18.6, 1)
sketch "Skizze3" plane through (0, 0, -2) normal (0, 0, -1) x (1, 0, 0)
  arc A0 (5.5129, -9.2) -> (5.3581, -9.6805) centre (7.7942, -10.2) ccw
  line L0 (5.5129, -9.2) -> (10.0756, -9.2)
  arc A1 (10.2304, -9.6805) -> (10.0756, -9.2) centre (7.7942, -10.2) ccw
  line L1 (10.2304, -9.6805) -> (13.1059, -4.7)
  line L2 (13.1059, -4.7) -> (18.302, -4.7)
  line L3 (18.302, -4.7) -> (20.9001, -0.2)
  line L4 (20.9001, -0.2) -> (26.0962, -0.2)
  line L5 (26.0962, -0.2) -> (28.8098, 4.5)
  line L6 (28.8098, 4.5) -> (26.2117, 9)
  line L7 (26.2117, 9) -> (28.8098, 13.5)
  line L8 (28.8098, 13.5) -> (26.2117, 18)
  line L9 (26.2117, 18) -> (28.8098, 22.5)
  line L10 (28.8098, 22.5) -> (26.0962, 27.2)
  line L11 (26.0962, 27.2) -> (20.9001, 27.2)
  line L12 (20.9001, 27.2) -> (18.302, 31.7)
  line L13 (18.302, 31.7) -> (13.1059, 31.7)
  line L14 (13.1059, 31.7) -> (10.5078, 36.2)
  line L15 (10.5078, 36.2) -> (5.0807, 36.2)
  line L16 (5.0807, 36.2) -> (2.4826, 31.7)
  line L17 (2.4826, 31.7) -> (-2.7135, 31.7)
  line L18 (-2.7135, 31.7) -> (-5.3116, 27.2)
  line L19 (-5.3116, 27.2) -> (-10.5078, 27.2)
  line L20 (-10.5078, 27.2) -> (-13.2213, 22.5)
  line L21 (-13.2213, 22.5) -> (-10.6232, 18)
  line L22 (-10.6232, 18) -> (-13.2213, 13.5)
  line L23 (-13.2213, 13.5) -> (-10.6232, 9)
  line L24 (-10.6232, 9) -> (-13.2213, 4.5)
  line L25 (-13.2213, 4.5) -> (-10.5078, -0.2)
  line L26 (-10.5078, -0.2) -> (-5.3116, -0.2)
  line L27 (-5.3116, -0.2) -> (-2.7135, -4.7)
  line L28 (-2.7135, -4.7) -> (2.4826, -4.7)
  line L29 (2.4826, -4.7) -> (5.3581, -9.6805)
  line L30 (15.5841, 17.9924) -> (15.5797, 18)
  line L31 (15.5797, 18) -> (15.5841, 18.0076)
  line L32 (15.5841, 18.0076) -> (15.5929, 18.0076)
  line L33 (15.5929, 18.0076) -> (15.5973, 18)
  line L34 (15.5973, 18) -> (15.5929, 17.9924)
  line L35 (15.5929, 17.9924) -> (15.5841, 17.9924)
  circle A2 centre (-6, 2.3) radius 0.75
  circle A3 centre (-3.1, 0.9) radius 0.75
  circle A4 centre (0, 0.3) radius 0.75
  circle A5 centre (4.5, 2.9) radius 0.75
  circle A6 centre (6.5, 0.9) radius 0.75
  circle A7 centre (9.9, 4.5) radius 0.75
  circle A8 centre (7.2, 6.4) radius 0.75
  circle A9 centre (23.9977, 19.3745) radius 0.75
  circle A10 centre (18, 20) radius 0.75
  circle A11 centre (14.536, 22.4075) radius 0.75
  circle A12 centre (10.8774, 25.0649) radius 0.75
  circle A13 centre (1.2415, 25.3138) radius 0.75
  circle A14 centre (3.1, 30.1) radius 0.75
  circle A15 centre (9.8, 29.1) radius 0.75
  line L36 (17.9556, 16.8725) -> (8.3956, 16.8453) construction
  line L37 (8.3956, 16.8453) -> (8.4096, 11.9214) construction
  line L38 (8.4096, 11.9214) -> (17.9695, 11.9485) construction
  line L39 (17.9695, 11.9485) -> (17.9556, 16.8725) construction
  line L40 (7.6275, 13.6111) -> (9.6045, 14.7525) construction
  line L41 (7.6275, 13.6111) -> (10.7308, 11.8195) construction
  line L42 (7.6275, 13.6111) -> (17.8333, 13.6111) construction
  arc A16 (4.7697, 15.2611) -> (4.7697, 11.9611) centre (7.6275, 13.6111) ccw
  arc A17 (2.6046, 16.5111) -> (2.6046, 10.7111) centre (7.6275, 13.6111) ccw
  arc A18 (0.4395, 17.7611) -> (0.4395, 9.4611) centre (7.6275, 13.6111) ccw
  arc A19 (6.9347, 14.0111) -> (6.9347, 13.2111) centre (7.6275, 13.6111) ccw
  arc A20 (5.8955, 14.6111) -> (5.8955, 12.6111) centre (7.6275, 13.6111) ccw
  arc A21 (3.7304, 15.8611) -> (3.7304, 11.3611) centre (7.6275, 13.6111) ccw
  arc A22 (1.5654, 17.1111) -> (1.5654, 10.1111) centre (7.6275, 13.6111) ccw
  arc A23 (-0.5997, 18.3611) -> (-0.5997, 8.8611) centre (7.6275, 13.6111) ccw
  line L43 (0.4395, 9.4611) -> (-0.5997, 8.8611) construction
  line L44 (1.5654, 10.1111) -> (2.6046, 10.7111) construction
  line L45 (3.7304, 11.3611) -> (4.7697, 11.9611) construction
  line L46 (5.8955, 12.6111) -> (6.9347, 13.2111) construction
  line L47 (6.9347, 14.0111) -> (5.8955, 14.6111) construction
  line L48 (4.7697, 15.2611) -> (3.7304, 15.8611) construction
  line L49 (2.6046, 16.5111) -> (1.5654, 17.1111) construction
  line L50 (0.4395, 17.7611) -> (-0.5997, 18.3611) construction
  arc A24 (5.8955, 12.6111) -> (6.9347, 13.2111) centre (6.3776, 12.976) ccw
  arc A25 (3.7304, 11.3611) -> (4.7697, 11.9611) centre (4.25, 11.6611) ccw
  arc A26 (1.5635, 10.1143) -> (2.6046, 10.7111) centre (2.085, 10.4111) ccw
  arc A27 (-0.5997, 8.8611) -> (0.4395, 9.4611) centre (-0.0801, 9.1611) ccw
  arc A28 (6.9347, 14.0111) -> (5.8955, 14.6111) centre (6.4151, 14.3111) ccw
  arc A29 (4.7697, 15.2611) -> (3.7304, 15.8611) centre (4.25, 15.5611) ccw
  arc A30 (2.6046, 16.5111) -> (1.5654, 17.1111) centre (2.085, 16.8111) ccw
  arc A31 (0.4395, 17.7611) -> (-0.5997, 18.3611) centre (-0.0801, 18.0611) ccw
  line L51 (7.7942, -9.2) -> (7.7942, 36.2) construction
  point P0 (7.6275, 13.6111)
  point P1 (6.4151, 14.3111)
  point P2 (4.25, 15.5611)
  point P3 (2.085, 16.8111)
  point P4 (-0.0801, 18.0611)
  point P5 (-0.0801, 9.1611)
  point P6 (2.085, 10.4111)
  point P7 (4.25, 11.6611)
  point P8 (6.4151, 12.9111)
  point P9 (6.9347, 13.2111)
  point P10 (5.8955, 12.6111)
  point P11 (4.7697, 11.9611)
  point P12 (3.7304, 11.3611)
  point P13 (2.6046, 10.7111)
  point P14 (1.5654, 10.1111)
  point P15 (0.4395, 9.4611)
  point P16 (-0.5997, 8.8611)
  dimension "d25" = 1.5
  dimension "d26" = 3.5
  dimension "d28" = 150
  dimension "d29" = 150
  dimension "d30" = 1.2
  dimension "d31" = 1.2
  dimension "d32" = 1.2
  dimension "d33" = 1.2
  dimension "d34" = 0.8
  dimension "d35" = 3.3
  dimension "d36" = 5.8
  dimension "d37" = 8.3
  text T0 "NFC" font "Arial" height 3.5 align left top in box 9.56 x 4.924 at (17.9556, 16.8725) x (-0.999996, -0.002841) y (0.002841, -0.999996) spacing 1 kerned
  constraint equal A2 A3
  constraint equal A3 A4
  constraint equal A4 A5
  constraint equal A5 A8
  constraint equal A7 A8
  constraint equal A6 A7
  constraint equal A2 A13
  constraint equal A13 A14
  constraint equal A14 A15
  constraint equal A12 A15
  constraint equal A11 A12
  constraint equal A10 A11
  constraint equal A9 A10
  constraint coincident P0 L40.start
  constraint horizontal L42
  constraint coincident L40 P11
  constraint coincident L40 P13
  constraint coincident L40 P15
  constraint coincident L40 P9
  constraint coincident L40 P10
  constraint coincident L40 P12
  constraint coincident L40 P14
  constraint coincident L40 P16
  constraint coincident L41 A19.start
  constraint coincident L41 A20.start
  constraint coincident L41 A16.start
  constraint coincident L41 A21.start
  constraint coincident L41 A17.start
  constraint coincident L41 A22.start
  constraint coincident L41 A18.start
  constraint coincident L41 A23.start
  constraint coincident P9 A19.end
  constraint coincident P10 A20.end
  constraint coincident P11 A16.end
  constraint coincident P12 A21.end
  constraint coincident P13 A17.end
  constraint coincident P14 A22.end
  constraint coincident P15 A18.end
  constraint coincident P16 A23.end
  constraint midpoint P1 L47
  constraint midpoint P2 L48
  constraint midpoint P3 L49
  constraint midpoint P4 L50
  constraint midpoint P5 L43
  constraint midpoint P6 L44
  constraint midpoint P7 L45
  constraint midpoint P8 L46
  constraint coincident P7 A25.centre
  constraint coincident P6 A26.centre
  constraint coincident P1 A28.centre
  constraint coincident P2 A29.centre
  constraint coincident P3 A30.centre
  constraint coincident P4 A31.centre
  constraint coincident P5 A27.centre
  constraint midpoint L0 L51.start
  constraint midpoint L15 L51.end
  measures "d25" diameter of A2
  measures "d28" angle of L40 L42
  measures "d29" angle of L41 L42
  measures "d30" distance of A19 A20
  measures "d31" distance of A16 A21
  measures "d32" distance of A17 A22
  measures "d33" distance of A18 A23
  measures "d34" distance of P0 P9
  measures "d35" distance of P11 P0
  measures "d36" distance of P0 P13
  measures "d37" distance of P0 P15
extrude "Extrusion5" cut sketch "Skizze3" sketch "Skizze3" against normal blind 0.1 contours A2 | A3 | A4 | A5 | A6 | A7 | A8 | A9 | A10 | A11 | A12 | A13 | A14 | A15 | A16 A21 A25 A29 | A17 A22 A26 A30 | A18 A23 A27 A31 | A19 A20 A24 A28 of sketch 2 text T0
equation "d2 = d1 - 1.2 mm"
equation "d3 = ( d1 - d2 - 0 mm ) * 1.5 - ( d1 - d2 ) / 2"
equation "d12 = d1"
equation "d29 = d28"
equation "d31 = d30"
equation "d32 = d30"
equation "d33 = d30"
equation "d35 = d34 + 2.5 mm"
equation "d36 = d35 + 2.5 mm"
equation "d37 = d36 + 2.5 mm"
